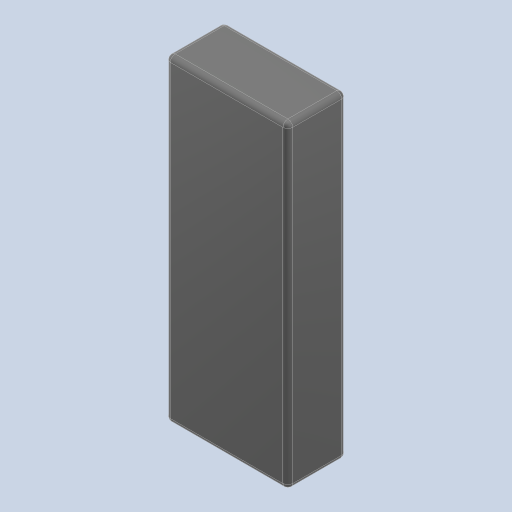
# Autodesk Inventor part: LiPo_800mAh
Saved by Autodesk Inventor 2023 (Build 270158000, 158)
## iProperties
Created: 2022-08-11
Part Number: LiPo_800mAh
Material: Acetal Resin, Black
Document SubType Name: Modeling
Designer: Windows10
Density: 1.425 g/cm^3
Appearance: Smooth - Black
Author: Windows10
Autodesk Inventor part; units mm, degrees
ref_plane "YZ Plane" through (0, 0, 0) normal (1, 0, 0) x (0, 1, 0)
ref_plane "XZ Plane" through (0, 0, 0) normal (0, 1, 0) x (-1, 0, 0)
ref_plane "XY Plane" through (0, 0, 0) normal (0, 0, 1) x (1, 0, 0)
sketch "Sketch1" plane through (0, 0, 0) normal (0, 0, 1) x (1, 0, 0)
  line L0 (0, 0) -> (25, 0)
  line L1 (25, 0) -> (25, -65)
  line L2 (25, -65) -> (0, -65)
  line L3 (0, -65) -> (0, 0)
  dimension "d0" = 25
  dimension "d1" = 65
  constraints: 8 end point, 2 parallel, 1 horizontal, 1 perpendicular
  measures "d0" distance of L1.end L2.end
  measures "d1" distance of L0.end L1.end
extrude "Extrusion1" add sketch "Sketch1" along normal blind 12
fillet "Fillet3" radius 1 12 edges at (25, -32.5, 0) (0, -32.5, 0) (0, -32.5, 12) (25, -32.5, 12) (12.5, 0, 0) (12.5, 0, 12) (0, 0, 6) (25, 0, 6) (12.5, -65, 0) (25, -65, 6) (0, -65, 6) (12.5, -65, 12)
body "Solid1"
